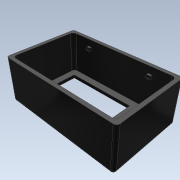
# Autodesk Inventor part: PT-00000024
Saved by Autodesk Inventor 2020.1 (Build 241239000, 239)
## iProperties
Created: 2020-06-15
Part Number: PT-00000024
Material: ABS Plastic
Document SubType Name: Modeling
Designer: Lance Haynie
Density: 1.06 g/cm^3
Appearance: Glossy - Black
Mass: 19.4441 g
Surface Area: 158.613 cm^2
Volume: 18.3435 cm^3
Engineer: Lance Haynie
Company: Haynie Research & Development, LLC
Author: HAYNIE
Autodesk Inventor part; units mm, degrees
ref_plane "YZ Plane" through (0, 0, 0) normal (1, 0, 0) x (0, 1, 0)
ref_plane "XZ Plane" through (0, 0, 0) normal (0, 1, 0) x (-1, 0, 0)
ref_plane "XY Plane" through (0, 0, 0) normal (0, 0, 1) x (1, 0, 0)
sketch "Box-Sketch" plane through (0, 0, 0) normal (0, 1, 0) x (-1, 0, 0)
  line L0 (37.5, -25) -> (37.5, 25)
  line L1 (37.5, 25) -> (-42.5, 25)
  line L2 (-42.5, 25) -> (-42.5, -25)
  line L3 (-42.5, -25) -> (37.5, -25)
  line L4 (37.5, 1.9049) -> (-42.5, 1.9049)
  point P0 (0, 0)
  dimension "d0" = 50
  dimension "d1" = 80
  dimension "d164" = 25
  dimension "d165" = 37.5
  constraints: 10 end point, 2 parallel, 2 perpendicular, 2 point on line
  measures "d0" distance of L2.end L1.end
  measures "d1" distance of L1.end L0.end
  measures "d164" distance from line of point (0, 0) L3
  measures "d165" distance from line of point (0, 0) L0
extrude "Box-Extrude" add sketch "Box-Sketch" along normal blind 30
shell "Box-Shell" thickness 2.5 removed faces 1 at (15.8333, 30, 8.3333)
sketch "LCD-Sketch" plane through (-35, 2.5, -22.5) normal (0, 1, 0) x (0, 0, 1)
  line L0 (5, 5) -> (40, 5)
  line L1 (40, 5) -> (40, 52.5)
  line L2 (40, 52.5) -> (5, 52.5)
  line L3 (5, 52.5) -> (5, 5)
  line L4 (0, 0) -> (0, 75) projected
  line L5 (45, 0) -> (0, 0) projected
  line L6 (45, 75) -> (45, 0) projected
  line L7 (-2.5, 77.5) -> (-2.5, -2.5) projected
  point P0 (22.5, 35)
  dimension "d41" = 35
  dimension "d42" = 47.5
  dimension "d160" = 5
  dimension "d166" = 17.5
  dimension "d167" = 17.5
  dimension "d168" = 5
  constraints: 8 end point, 2 parallel, 1 horizontal, 1 perpendicular
  measures "d41" distance of L2.end L1.end
  measures "d42" distance of L1.end L0.end
  measures "d160" distance between parallel lines of L5 L0
  measures "d166" distance from line of L3 point (22.5, 35)
  measures "d167" distance from line of L1 point (22.5, 35)
  measures "d168" distance between parallel lines of L4 L3
extrude "LCD-Extrude" cut sketch "LCD-Sketch" against normal up to next
fillet "Fillet1" radius 2 1 edges at (42.5, 0, 0)
fillet "Fillet2" radius 2 3 edges at (1.5, 0, -25) (41.9142, 0.5858, -25) (42.5, 16, -25)
fillet "Fillet3" radius 2 3 edges at (1.5, 0, 25) (41.9142, 0.5858, 25) (42.5, 16, 25)
fillet "Fillet4" radius 2 5 edges at (-37.5, 0, 0) (-37.5, 0.5858, 24.4142) (-37.5, 16, 25) (-37.5, 0.5858, -24.4142) (-37.5, 16, -25)
fillet "Fillet5" radius 2.5 1 edges at (-35, 16.25, -22.5)
fillet "Fillet6" radius 2.5 1 edges at (40, 16.25, 22.5)
fillet "Fillet7" radius 2.5 1 edges at (-35, 16.25, 22.5)
fillet "Fillet8" radius 2.5 1 edges at (40, 16.25, -22.5)
sketch "Sketch16" plane through (37.5, 2.5, 22.5) normal (0, 0, -1) x (-1, 0, 0)
  line L0 (56, 20) -> (59, 20) projected
  line L1 (56, 23) -> (56, 20) projected
  line L2 (59, 23) -> (56, 23) projected
  line L3 (60, 20) -> (60, 23) projected
  line L4 (59, 20) -> (56, 20)
  line L5 (56, 20) -> (56, 23)
  line L6 (56, 23) -> (59, 23)
  line L7 (59, 23) -> (59, 20)
  line L8 (11, 20) -> (14, 20) projected
  line L9 (10.5, 23) -> (10.5, 20) projected
  line L10 (14, 23) -> (11, 23) projected
  line L11 (14, 20) -> (14, 23) projected
  line L12 (14, 20) -> (11, 20)
  line L13 (11, 20) -> (11, 23)
  line L14 (11, 23) -> (14, 23)
  line L15 (14, 23) -> (14, 20)
  line L16 (58.75, 20.25) -> (56.25, 20.25)
  line L17 (56.25, 20.25) -> (56.25, 22.75)
  line L18 (56.25, 22.75) -> (58.75, 22.75)
  line L19 (58.75, 22.75) -> (58.75, 20.25)
  line L20 (58.75, 20.25) -> (56.25, 22.75) construction
  line L21 (56.25, 20.25) -> (58.75, 22.75) construction
  line L22 (13.75, 20.25) -> (11.25, 20.25)
  line L23 (11.25, 20.25) -> (11.25, 22.75)
  line L24 (11.25, 22.75) -> (13.75, 22.75)
  line L25 (13.75, 22.75) -> (13.75, 20.25)
  line L26 (13.75, 20.25) -> (11.25, 22.75) construction
  line L27 (11.25, 20.25) -> (13.75, 22.75) construction
  line L28 (73, 27.5) -> (-3, 27.5) projected
  point P0 (37.5, -2.5)
  point P1 (57.5, 21.5)
  point P2 (12.5, 21.5)
  dimension "d232" = 2.5
  dimension "d233" = 2.5
  dimension "d234" = 2.5
  dimension "d235" = 2.5
  dimension "d250" = 4.75
  dimension "d251" = 4.75
  constraints: 40 end point, 8 parallel, 4 horizontal, 4 midpoint, 4 perpendicular
  measures "d232" distance of L17.end L18.end
  measures "d233" distance of L16.end L17.end
  measures "d234" distance of L23.end L24.end
  measures "d235" distance of L22.end L23.end
  measures "d250" distance between parallel lines of L28 L24
  measures "d251" distance between parallel lines of L28 L18
extrude "Extrusion10" add sketch "Sketch16" along normal blind 2.5 contours L16 L17 L18 L19 | L22 L23 L24 L25
chamfer "Chamfer9" distance 1 angle 45 4 edges at (-20, 25.25, 20) (25, 25.25, 20) (-20, 22.75, 20) (25, 22.75, 20)
sketch "Sketch17" plane through (-32.5, 2.5, -22.5) normal (0, 0, 1) x (1, 0, 0)
  line L0 (56, 20) -> (59, 20) projected
  line L1 (56, 23) -> (56, 20) projected
  line L2 (59, 23) -> (56, 23) projected
  line L3 (59, 20) -> (59, 23) projected
  line L4 (58.75, 20.25) -> (56.25, 20.25)
  line L5 (56.25, 20.25) -> (56.25, 22.75)
  line L6 (56.25, 22.75) -> (58.75, 22.75)
  line L7 (58.75, 22.75) -> (58.75, 20.25)
  line L8 (58.75, 20.25) -> (56.25, 22.75) construction
  line L9 (56.25, 20.25) -> (58.75, 22.75) construction
  line L10 (11, 20) -> (14, 20) projected
  line L11 (11, 23) -> (11, 20) projected
  line L12 (14, 23) -> (11, 23) projected
  line L13 (14, 20) -> (14, 23) projected
  line L14 (13.75, 20.25) -> (11.25, 20.25)
  line L15 (11.25, 20.25) -> (11.25, 22.75)
  line L16 (11.25, 22.75) -> (13.75, 22.75)
  line L17 (13.75, 22.75) -> (13.75, 20.25)
  line L18 (13.75, 20.25) -> (11.25, 22.75) construction
  line L19 (11.25, 20.25) -> (13.75, 22.75) construction
  line L20 (-3, 27.5) -> (73, 27.5) projected
  point P0 (32.5, -2.5)
  point P1 (57.5, 21.5)
  point P2 (12.5, 21.5)
  dimension "d241" = 2.5
  dimension "d242" = 2.5
  dimension "d243" = 2.5
  dimension "d244" = 2.5
  dimension "d252" = 4.75
  dimension "d253" = 4.75
  constraints: 24 end point, 4 midpoint, 4 parallel, 2 horizontal, 2 perpendicular
  measures "d241" distance of L5.end L6.end
  measures "d242" distance of L4.end L5.end
  measures "d243" distance of L15.end L16.end
  measures "d244" distance of L14.end L15.end
  measures "d252" distance between parallel lines of L20 L6
  measures "d253" distance between parallel lines of L20 L16
extrude "Extrusion11" add sketch "Sketch17" along normal blind 2.5 contours L4 L5 L6 L7 | L14 L15 L16 L17
chamfer "Chamfer10" distance 1 angle 45 4 edges at (25, 25.25, -20) (25, 22.75, -20) (-20, 22.75, -20) (-20, 25.25, -20)
sketch "Sketch20" plane through (0, 0, 0) normal (0, -1, 0) x (1, 0, 0)
  line L0 (17.5, 17.5) -> (17.5, -17.5) projected
  line L1 (40.5, 23) -> (40.5, -23) projected
  line L2 (17.5, -17.5) -> (-30, -17.5) projected
  line L3 (-30, 17.5) -> (17.5, 17.5) projected
  point P0 (0, 0)
  point P1 (29, 0)
  dimension "d254" = 11.5
  dimension "d255" = 11.5
  dimension "d256" = 17.5
  dimension "d257" = 17.5
  measures "d254" distance from line of point (29, 0) L0
  measures "d255" distance from line of L1 point (29, 0)
  measures "d256" distance from line of L2 point (29, 0)
  measures "d257" distance from line of L3 point (29, 0)
hole "Hole12" at (29, 0, 0) direction (0, 1, 0) diameter 5 end through all
body "Solid1"
